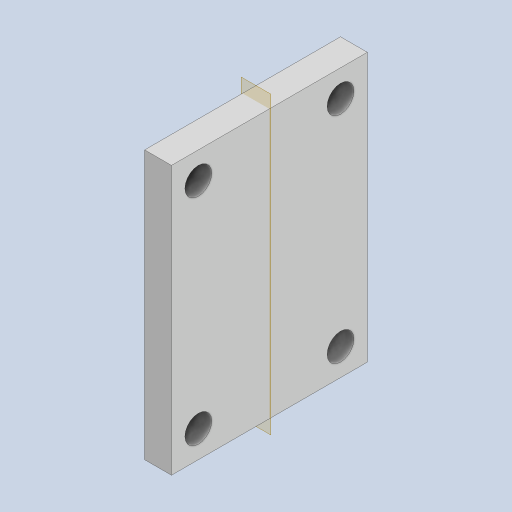
# Autodesk Inventor part: держатель магнитов на основе
Saved by Autodesk Inventor 2024.2 (Build 282272000, 272)
## iProperties
Created: 2025-12-27
Part Number: держатель магнитов на основе
Material: Типовые
Document SubType Name: Modeling
Designer: katya_notebook
Density: 1 g/cm^3
Appearance: По умолчанию
Author: katya_notebook
Autodesk Inventor part; units mm, degrees
ref_plane "YZ Plane" through (0, 0, 0) normal (1, 0, 0) x (0, 1, 0)
ref_plane "XZ Plane" through (0, 0, 0) normal (0, 1, 0) x (-1, 0, 0)
sketch "Эскиз1" plane through (0, 0, 0) normal (1, 0, 0) x (0, 1, 0)
  line L0 (-15, -10.95) -> (15, -10.95)
  line L1 (15, -10.95) -> (15, 10.95)
  line L2 (15, 10.95) -> (-15, 10.95)
  line L3 (-15, 10.95) -> (-15, -10.95)
  line L4 (-15, -10.95) -> (15, 10.95) construction
  line L5 (15, -10.95) -> (-15, 10.95) construction
  circle A0 centre (7, 0) radius 5
  circle A1 centre (-7, 0) radius 5
  point P0 (0, 0)
  dimension "d0" = 30
  dimension "d1" = 21.9
  dimension "d2" = 10
  dimension "d3" = 10
  dimension "d4" = 8
  dimension "d5" = 14
  dimension "d6" = 8
  dimension "d7" = 0
  constraints: 12 end point, 2 centre point, 2 midpoint, 2 parallel, 1 horizontal, 1 perpendicular
  measures "d0" distance of L1.end L2.end
  measures "d1" distance of L0.end L1.end
  measures "d2" diameter of A0
  measures "d3" diameter of A1
  measures "d4" distance from line of A0.centre L1
  measures "d5" distance of A1.centre A0.centre
  measures "d6" distance from line of L3 A1.centre
  measures "d7" vertical distance of point (0, 0) A0.centre
extrude "Выдавливание1" add sketch "Эскиз1" along normal blind 2
sketch "Эскиз2" plane through (2, 0, 0) normal (1, 0, 0) x (0, 0, -1)
  line L0 (10.95, 15) -> (-10.95, 15) projected
  line L1 (10.95, -15) -> (-10.95, -15)
  line L2 (-10.95, -15) -> (-10.95, 15)
  line L3 (-10.95, 15) -> (10.95, 15)
  line L4 (10.95, 15) -> (10.95, -15)
  line L5 (10.95, -15) -> (-10.95, 15) construction
  line L6 (-10.95, -15) -> (10.95, 15) construction
  point P0 (0, 0)
  constraints: 12 end point, 2 midpoint, 2 parallel, 1 horizontal, 1 perpendicular
extrude "Выдавливание2" add sketch "Эскиз2" along normal blind 1
sketch "Эскиз3" plane through (0, 0, 0) normal (-1, 0, 0) x (0, 0, 1)
  circle A0 centre (-7.95, 12) radius 1.5
  line L0 (-10.95, 15) -> (10.95, 15) projected
  line L1 (-10.95, -15) -> (-10.95, 15) projected
  circle A1 centre (-7.95, -12) radius 1.5
  line L2 (10.95, -15) -> (-10.95, -15) projected
  circle A2 centre (7.95, 12) radius 1.5
  line L3 (10.95, 15) -> (10.95, -15) projected
  circle A3 centre (7.95, -12) radius 1.5
  point P0 (0, 0)
  dimension "d12" = 3
  dimension "d13" = 3
  dimension "d14" = 3
  dimension "d15" = 3
  dimension "d16" = 3
  dimension "d17" = 3
  dimension "d18" = 3
  dimension "d19" = 3
  dimension "d20" = 3
  constraints: 4 centre point
  measures "d12" diameter of A0
  measures "d13" distance from line of L0 A0.centre
  measures "d14" distance from line of L1 A0.centre
  measures "d15" diameter of A1
  measures "d16" distance from line of L1 A1.centre
  measures "d17" distance from line of L2 A1.centre
  measures "d18" diameter of A2
  measures "d19" distance from line of L3 A2.centre
  measures "d20" diameter of A3
extrude "Выдавливание3" cut sketch "Эскиз3" against normal blind 3 contours A0 | A1 | A2 | A3
